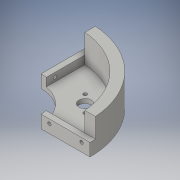
# Autodesk Inventor part: base_segment
Saved by Autodesk Inventor 2016 (Build 200138000, 138)
## iProperties
Created: 2016-02-27
Part Number: base_segment
Material: Generic
Document SubType Name: Modeling
Designer: Matt Ruffner
Density: 1 g/cm^3
Appearance: Default
Author: Matt Ruffner
Autodesk Inventor part; units mm, degrees
ref_plane "YZ Plane" through (0, 0, 0) normal (1, 0, 0) x (0, 1, 0)
ref_plane "XZ Plane" through (0, 0, 0) normal (0, 1, 0) x (-1, 0, 0)
ref_plane "XY Plane" through (0, 0, 0) normal (0, 0, 1) x (1, 0, 0)
sketch "Sketch1" plane through (0, 0, 0) normal (0, 1, 0) x (-1, 0, 0)
  arc A0 (-76.2, 0) -> (0, -76.2) centre (0, 0) ccw
  line L0 (-76.2, 0) -> (-31.75, 0)
  line L1 (0, -76.2) -> (0, -31.75)
  arc A1 (-31.75, 0) -> (0, -31.75) centre (0, 0) ccw
  line L2 (0, 0) -> (-35.921, -35.921)
  line L3 (0, 0) -> (50.8, 0) construction
  circle A2 centre (-35.921, -35.921) radius 5.715
  line L4 (-35.921, -35.921) -> (-28.5572, -43.2848)
  line L5 (-35.921, -35.921) -> (-25.507, -35.921) construction
  line L6 (-35.921, -35.921) -> (-43.2848, -28.5572)
  circle A3 centre (-28.5572, -43.2848) radius 1.651
  circle A4 centre (-43.2848, -28.5572) radius 1.651
  dimension "d0" = 152.4
  dimension "d1" = 44.45
  dimension "d2" = 44.45
  dimension "d3" = 50.8
  dimension "d4" = 135
  dimension "d5" = 11.43
  dimension "d6" = 10.414
  dimension "d7" = 45
  dimension "d8" = 10.414
  dimension "d9" = 3.302
  dimension "d10" = 3.302
  constraints: 14 end point, 5 centre point, 5 coincident, 4 point on circle, 3 horizontal, 2 equal length, 1 vertical
  measures "d0" diameter of A0
  measures "d1" distance of L0.start L0.end
  measures "d2" distance of L1.end L1.start
  measures "d3" distance of L2.start L2.end
  measures "d4" angle of L2 L3
  measures "d5" diameter of A2
  measures "d6" distance of L4.start L4.end
  measures "d7" angle of L4 L5
  measures "d8" distance of L4.start L6.end
  measures "d9" diameter of A3
  measures "d10" diameter of A4
extrude "Extrusion1" add sketch "Sketch1" along normal blind 3.937
sketch "Sketch4" plane through (0, 3.937, 0) normal (0, 1, 0) x (1, 0, 0)
  circle A0 centre (35.921, 35.921) radius 5.715 projected
  circle A1 centre (43.2848, 28.5572) radius 1.651 projected
  circle A2 centre (28.5572, 43.2848) radius 1.651 projected
  arc A3 (76.2, 0) -> (0, 76.2) centre (0, 0) ccw projected
  line L0 (0, 76.2) -> (0, 31.75) projected
  arc A4 (31.75, 0) -> (0, 31.75) centre (0, 0) ccw projected
  line L1 (31.75, 0) -> (76.2, 0) projected
  line L2 (5.08, 76.0305) -> (5.08, 31.341)
  line L3 (31.341, 5.08) -> (76.0305, 5.08)
  dimension "d15" = 5.08
  dimension "d16" = 5.08
  constraints: 4 end point, 4 point on circle, 1 horizontal, 1 vertical
  measures "d15" distance between parallel lines of L1 L3
  measures "d16" distance between parallel lines of L0 L2
extrude "Extrusion2" add sketch "Sketch4" along normal blind 7.62 contours L1 A4 L3 A3 | L2 A4 L0 A3
sketch "Sketch5" plane through (31.75, 0, 0) normal (0, 0, 1) x (1, 0, 0)
  line L0 (0, 0) -> (0, 11.557) projected
  line L1 (0, 7.747) -> (44.3964, 7.747)
  line L2 (0, 11.557) -> (44.45, 11.557) projected
  circle A0 centre (7.62, 7.747) radius 1.524
  circle A1 centre (36.83, 7.747) radius 1.524
  line L3 (44.45, 0) -> (44.45, 11.557) projected
  point P0 (-31.75, 0)
  dimension "d19" = 3.81
  dimension "d20" = 3.048
  dimension "d21" = 3.048
  dimension "d22" = 7.62
  dimension "d23" = 7.62
  constraints: 3 point on line, 2 centre point, 2 end point, 1 horizontal
  measures "d19" distance between parallel lines of L2 L1
  measures "d20" diameter of A0
  measures "d21" diameter of A1
  measures "d22" distance of L1.start A0.centre
  measures "d23" distance from line of L3 A1.centre
extrude "Extrusion3" cut sketch "Sketch5" against normal through all
sketch "Sketch6" plane through (0, 0, -76.2) normal (-1, 0, 0) x (0, 0, 1)
  line L0 (0.0164, 7.747) -> (43.8758, 7.747)
  line L1 (0, 11.557) -> (44.45, 11.557) projected
  circle A0 centre (7.6364, 7.747) radius 1.524
  circle A1 centre (36.83, 7.747) radius 1.524
  line L2 (44.45, 0) -> (44.45, 11.557) projected
  point P0 (76.2, 0)
  dimension "d26" = 3.81
  dimension "d27" = 3.048
  dimension "d28" = 3.048
  dimension "d29" = 7.62
  dimension "d30" = 7.62
  constraints: 2 centre point, 2 end point, 2 point on line, 1 horizontal
  measures "d26" distance between parallel lines of L1 L0
  measures "d27" diameter of A0
  measures "d28" diameter of A1
  measures "d29" distance of L0.start A0.centre
  measures "d30" distance from line of L2 A1.centre
extrude "Extrusion4" cut sketch "Sketch6" against normal blind 7.62
sketch "Sketch7" plane through (0, 3.937, 0) normal (0, 1, 0) x (1, 0, 0)
  arc A0 (76.0305, 5.08) -> (5.08, 76.0305) centre (0, 0) ccw projected
  line L0 (5.08, 31.341) -> (5.08, 76.0305) projected
  line L1 (76.0305, 5.08) -> (31.341, 5.08) projected
  arc A1 (66.4812, 5.08) -> (5.08, 66.4812) centre (0, 0) ccw
  dimension "d33" = 133.35
  constraints: 2 point on circle, 2 point on line, 1 centre point, 1 coincident
  measures "d33" diameter of A1
extrude "Extrusion5" add sketch "Sketch7" along normal blind 25.4
body "Solid1"
